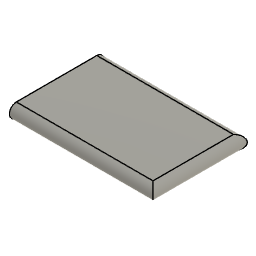
WatchAssembly v8 (Autodesk Fusion 360 archive; units mm, degrees)
design "LiPo_BlockIn"
Autodesk Fusion 360 part; units mm, degrees
sketch "Sketch1" plane through (0, 0, 0) normal (0, 0, 1) x (1, 0, 0) in component "RD-1342_LiPo_3.7_1100mAh"
  line L0 (0, 0) -> (52, 0)
  line L1 (52, 0) -> (52, 34)
  line L2 (52, 34) -> (0, 34)
  line L3 (0, 34) -> (0, 0)
  dimension "d1" = 52
  dimension "d2" = 34
  constraint horizontal L0
  constraint vertical L1
  constraint horizontal L2
  constraint vertical L3
  constraint coincident L0.start L3.end
  measures "d1" distance of L0.start L0.end
  measures "d2" distance of L0.start L2.end
extrude "Extrude1" add sketch "Sketch1" along normal blind 5 in component "RD-1342_LiPo_3.7_1100mAh"
fillet "Fillet1" radius 2.5 6 edges at (26, 34, 5) (26, 0, 5) (52, 17, 5) (52, 17, 0) (26, 34, 0) (26, 0, 0) in component "RD-1342_LiPo_3.7_1100mAh"
sketch "Sketch2" plane through (0, 0, 0) normal (-1, 0, 0) x (0, -1, 0) in component "RD-1342_LiPo_3.7_1100mAh"
  arc A0 (-31.5, 5) -> (-31.5, 0) centre (-31.5, 2.5) ccw
  line L0 (-31.5, 0) -> (-2.5, 0)
  arc A1 (-2.5, 0) -> (-2.5, 5) centre (-2.5, 2.5) ccw
  line L1 (-2.5, 5) -> (-31.5, 5)
  line L2 (-31.5, 0.5) -> (-2.5, 0.5)
  arc A2 (-2.5, 0.5) -> (-2.5, 4.5) centre (-2.5, 2.5) ccw
  line L3 (-2.5, 4.5) -> (-31.5, 4.5)
  arc A3 (-31.5, 4.5) -> (-31.5, 0.5) centre (-31.5, 2.5) ccw
  dimension "d7" = -0.5
extrude "Extrude2" cut sketch "Sketch2" against normal blind 4 contours L2 A2 L3 A3 in component "RD-1342_LiPo_3.7_1100mAh"
fillet "Fillet2" radius 2 1 faces at (4, 21.8333, 3.1667) in component "RD-1342_LiPo_3.7_1100mAh"
fillet "Fillet3" radius 0.25 1 faces at (0, 12.1667, 0.1667) in component "RD-1342_LiPo_3.7_1100mAh"
component "RD-1342_LiPo_3.7_1100mAh" placed x (1, 0, 0) y (0, 1, 0) z (0, 0, 1) at (0, 0, 0)
